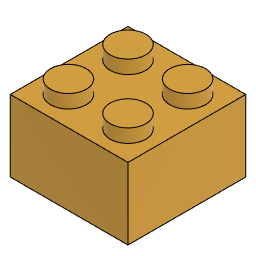
Yellow 2x2 (Autodesk Fusion 360 design; units mm, degrees)
Autodesk Fusion 360 part; units mm, degrees
sketch "Sketch1" plane through (0, 0, 0) normal (0, 0, 1) x (1, 0, 0)
  line L0 (0, 0) -> (15.8, 0)
  line L1 (15.8, 0) -> (15.8, 15.8)
  line L2 (15.8, 15.8) -> (0, 15.8)
  line L3 (0, 15.8) -> (0, 0)
  circle A0 centre (3.9, 11.9) radius 2.4
  circle A1 centre (11.9, 11.9) radius 2.4
  circle A2 centre (11.9, 3.9) radius 2.4
  circle A3 centre (3.9, 3.9) radius 2.4
  line L4 (1.2, 1.2) -> (14.6, 1.2)
  line L5 (14.6, 1.2) -> (14.6, 14.6)
  line L6 (14.6, 14.6) -> (1.2, 14.6)
  line L7 (1.2, 14.6) -> (1.2, 1.2)
  circle A4 centre (7.9, 7.9) radius 3.255
  circle A5 centre (7.9, 7.9) radius 2.4
  circle A6 centre (3.9, 11.9) radius 1.3
  circle A7 centre (11.9, 11.9) radius 1.3
  circle A8 centre (11.9, 3.9) radius 1.3
  circle A9 centre (3.9, 3.9) radius 1.3
  dimension "d1" = 15.8
  dimension "d2" = 15.8
  dimension "d3" = 4.8
  dimension "d4" = 4.8
  dimension "d5" = 4.8
  dimension "d6" = 4.8
  dimension "d7" = 8
  dimension "d8" = 8
  dimension "d9" = 8
  dimension "d10" = 8
  dimension "d11" = 3.9
  dimension "d12" = 3.9
  dimension "d13" = 3.9
  dimension "d14" = 13.4
  dimension "d15" = 13.4
  dimension "d16" = 1.2
  dimension "d17" = 1.2
  dimension "d18" = 6.51
  dimension "d19" = 6.7
  dimension "d20" = 6.7
  dimension "d21" = 4.8
  dimension "d22" = 2.6
  dimension "d23" = 2.6
  dimension "d24" = 2.6
  dimension "d25" = 2.6
  dimension "d32" = 3.9
  constraint horizontal L0
  constraint vertical L1
  constraint horizontal L2
  constraint vertical L3
  constraint coincident L0.start L3.end
  constraint horizontal L4
  constraint vertical L5
  constraint horizontal L6
  constraint vertical L7
  constraint concentric A4 A5
  constraint concentric A0 A6
  constraint concentric A1 A7
  constraint concentric A2 A8
  constraint concentric A3 A9
  measures "d1" distance of L0.start L0.end
  measures "d2" distance of L0.start L2.end
  measures "d3" diameter of A0
  measures "d4" diameter of A1
  measures "d5" diameter of A2
  measures "d6" diameter of A3
  measures "d7" horizontal distance of A2.centre A3.centre
  measures "d8" vertical distance of A0.centre A3.centre
  measures "d9" distance of A1.centre A2.centre
  measures "d10" horizontal distance of A0.centre A1.centre
  measures "d11" distance of L1 A2.centre
  measures "d12" distance of L2 A1.centre
  measures "d13" distance of L0 A3.centre
  measures "d14" distance of L4.start L4.end
  measures "d15" distance of L4.start L6.end
  measures "d16" distance of L3 L7
  measures "d17" distance of L0 L4
  measures "d18" diameter of A4
  measures "d19" distance of L5 A4.centre
  measures "d20" distance of L6 A4.centre
  measures "d21" diameter of A5
  measures "d22" diameter of A6
  measures "d23" diameter of A7
  measures "d24" diameter of A8
  measures "d25" diameter of A9
  measures "d32" distance of L0 A2.centre
extrude "Extrude1" add sketch "Sketch1" along normal blind 9.6 contours L0 L1 L2 L3 | A4 makes body 1 at (0, 10.5333, 3.2) makes body 2 at (11.1388, 8.2241, 6.4)
extrude "Extrude2" add sketch "Sketch1" along normal blind 9.6 and the other way blind -8.6 contours A0 | A1 | A2 | A3 | L4 L5 L6 L7 | A5 bodies 1 2
extrude "Extrude3" add sketch "Sketch1" along normal blind 11.4 and the other way blind -9.6 contours A0 | A1 | A2 | A3 | A6 | A7 | A8 | A9 bodies 1
extrude "Extrude4" cut sketch "Sketch1" along normal blind 10.3 contours A6 | A7 | A8 | A9 bodies 1
copy_body "Body->Comp1" bodies 1 removing the originals makes body 3 in component "Yellow 2x2"
component "Yellow 2x2" placed x (1, 0, 0) y (0, 1, 0) z (0, 0, 1) at (0, 0, 0)
equation "d14 = 15.8 mm - 1.2 mm - 1.2 mm"
equation "d15 = 15.8 mm - 1.2 mm - 1.2 mm"
equation "d19 = ( 13.4 / 2 ) * 1 mm"
equation "d33 = 9.6 mm + 1.8 mm"
equation "d37 = 9.6 mm + 0.7 mm"
named bodies: "Yellow 2x2"
